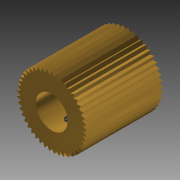
# Autodesk Inventor part: extruder_gear
Saved by Autodesk Inventor 2013 (Build 170138000, 138)
## iProperties
Created: 2015-02-21
Part Number: extruder_gear
Material: 一般
Document SubType Name: Modeling
Designer: Noa Izumi
Density: 1 g/cm^3
Author: Noa Izumi
Autodesk Inventor part; units mm, degrees
ref_plane "YZ Plane" through (0, 0, 0) normal (1, 0, 0) x (0, 1, 0)
ref_plane "XZ Plane" through (0, 0, 0) normal (0, 1, 0) x (-1, 0, 0)
ref_plane "XY Plane" through (0, 0, 0) normal (0, 0, 1) x (1, 0, 0)
sketch "草圖1" plane through (0, 0, 0) normal (0, 1, 0) x (-1, 0, 0)
  circle A0 centre (0, 0) radius 4.75
  line L0 (0, 5.5) -> (0.6495, 4.375)
  line L1 (0.6495, 4.375) -> (-0.6495, 4.375)
  line L2 (-0.6495, 4.375) -> (0, 5.5)
  line L3 (-0.7655, 5.4465) -> (0.0343, 4.4228)
  line L4 (0.0343, 4.4228) -> (-1.2521, 4.242)
  line L5 (-1.2521, 4.242) -> (-0.7655, 5.4465)
  line L6 (-1.516, 5.2869) -> (-0.5816, 4.3846)
  line L7 (-0.5816, 4.3846) -> (-1.8303, 4.0265)
  line L8 (-1.8303, 4.0265) -> (-1.516, 5.2869)
  line L9 (-2.2371, 5.0245) -> (-1.1861, 4.2609)
  line L10 (-1.1861, 4.2609) -> (-2.3728, 3.7326)
  line L11 (-2.3728, 3.7326) -> (-2.2371, 5.0245)
  line L12 (-2.9146, 4.6643) -> (-1.7676, 4.0544)
  line L13 (-1.7676, 4.0544) -> (-2.8692, 3.366)
  line L14 (-2.8692, 3.366) -> (-2.9146, 4.6643)
  line L15 (-3.5353, 4.2132) -> (-2.3146, 3.7689)
  line L16 (-2.3146, 3.7689) -> (-3.3098, 2.9339)
  line L17 (-3.3098, 2.9339) -> (-3.5353, 4.2132)
  line L18 (-4.0873, 3.6802) -> (-2.8166, 3.4101)
  line L19 (-2.8166, 3.4101) -> (-3.6859, 2.4448)
  line L20 (-3.6859, 2.4448) -> (-4.0873, 3.6802)
  line L21 (-4.5597, 3.0756) -> (-3.2638, 2.9849)
  line L22 (-3.2638, 2.9849) -> (-3.9902, 1.908)
  line L23 (-3.9902, 1.908) -> (-4.5597, 3.0756)
  line L24 (-4.9434, 2.411) -> (-3.6475, 2.5017)
  line L25 (-3.6475, 2.5017) -> (-4.217, 1.3341)
  line L26 (-4.217, 1.3341) -> (-4.9434, 2.411)
  line L27 (-5.2308, 1.6996) -> (-3.9602, 1.9697)
  line L28 (-3.9602, 1.9697) -> (-4.3616, 0.7342)
  line L29 (-4.3616, 0.7342) -> (-5.2308, 1.6996)
  line L30 (-5.4164, 0.9551) -> (-4.1957, 1.3994)
  line L31 (-4.1957, 1.3994) -> (-4.4213, 0.1201)
  line L32 (-4.4213, 0.1201) -> (-5.4164, 0.9551)
  line L33 (-5.4966, 0.1919) -> (-4.3497, 0.8018)
  line L34 (-4.3497, 0.8018) -> (-4.395, -0.4964)
  line L35 (-4.395, -0.4964) -> (-5.4966, 0.1919)
  line L36 (-5.4699, -0.5749) -> (-4.4189, 0.1886)
  line L37 (-4.4189, 0.1886) -> (-4.2831, -1.1033)
  line L38 (-4.2831, -1.1033) -> (-5.4699, -0.5749)
  line L39 (-5.3366, -1.3306) -> (-4.4022, -0.4282)
  line L40 (-4.4022, -0.4282) -> (-4.0879, -1.6886)
  line L41 (-4.0879, -1.6886) -> (-5.3366, -1.3306)
  line L42 (-5.0995, -2.0603) -> (-4.2997, -1.0367)
  line L43 (-4.2997, -1.0367) -> (-3.8131, -2.2411)
  line L44 (-3.8131, -2.2411) -> (-5.0995, -2.0603)
  line L45 (-4.7631, -2.75) -> (-4.1136, -1.625)
  line L46 (-4.1136, -1.625) -> (-3.4641, -2.75)
  line L47 (-3.4641, -2.75) -> (-4.7631, -2.75)
  line L48 (-4.3341, -3.3861) -> (-3.8474, -2.1817)
  line L49 (-3.8474, -2.1817) -> (-3.0477, -3.2053)
  line L50 (-3.0477, -3.2053) -> (-4.3341, -3.3861)
  line L51 (-3.8206, -3.9564) -> (-3.5064, -2.6959)
  line L52 (-3.5064, -2.6959) -> (-2.5719, -3.5983)
  line L53 (-2.5719, -3.5983) -> (-3.8206, -3.9564)
  line L54 (-3.2328, -4.4496) -> (-3.097, -3.1577)
  line L55 (-3.097, -3.1577) -> (-2.0461, -3.9212)
  line L56 (-2.0461, -3.9212) -> (-3.2328, -4.4496)
  line L57 (-2.5821, -4.8562) -> (-2.6274, -3.558)
  line L58 (-2.6274, -3.558) -> (-1.4804, -4.1678)
  line L59 (-1.4804, -4.1678) -> (-2.5821, -4.8562)
  line L60 (-1.8811, -5.1683) -> (-2.1067, -3.889)
  line L61 (-2.1067, -3.889) -> (-0.886, -4.3333)
  line L62 (-0.886, -4.3333) -> (-1.8811, -5.1683)
  line L63 (-1.1435, -5.3798) -> (-1.5449, -4.1444)
  line L64 (-1.5449, -4.1444) -> (-0.2743, -4.4144)
  line L65 (-0.2743, -4.4144) -> (-1.1435, -5.3798)
  line L66 (-0.3837, -5.4866) -> (-0.9531, -4.319)
  line L67 (-0.9531, -4.319) -> (0.3428, -4.4097)
  line L68 (0.3428, -4.4097) -> (-0.3837, -5.4866)
  line L69 (0.3837, -5.4866) -> (-0.3428, -4.4097)
  line L70 (-0.3428, -4.4097) -> (0.9531, -4.319)
  line L71 (0.9531, -4.319) -> (0.3837, -5.4866)
  line L72 (1.1435, -5.3798) -> (0.2743, -4.4144)
  line L73 (0.2743, -4.4144) -> (1.5449, -4.1444)
  line L74 (1.5449, -4.1444) -> (1.1435, -5.3798)
  line L75 (1.8811, -5.1683) -> (0.886, -4.3333)
  line L76 (0.886, -4.3333) -> (2.1067, -3.889)
  line L77 (2.1067, -3.889) -> (1.8811, -5.1683)
  line L78 (2.5821, -4.8562) -> (1.4804, -4.1678)
  line L79 (1.4804, -4.1678) -> (2.6274, -3.558)
  line L80 (2.6274, -3.558) -> (2.5821, -4.8562)
  line L81 (3.2328, -4.4496) -> (2.0461, -3.9212)
  line L82 (2.0461, -3.9212) -> (3.097, -3.1577)
  line L83 (3.097, -3.1577) -> (3.2328, -4.4496)
  line L84 (3.8206, -3.9564) -> (2.5719, -3.5983)
  line L85 (2.5719, -3.5983) -> (3.5064, -2.6959)
  line L86 (3.5064, -2.6959) -> (3.8206, -3.9564)
  line L87 (4.3341, -3.3861) -> (3.0477, -3.2053)
  line L88 (3.0477, -3.2053) -> (3.8474, -2.1817)
  line L89 (3.8474, -2.1817) -> (4.3341, -3.3861)
  line L90 (4.7631, -2.75) -> (3.4641, -2.75)
  line L91 (3.4641, -2.75) -> (4.1136, -1.625)
  line L92 (4.1136, -1.625) -> (4.7631, -2.75)
  line L93 (5.0995, -2.0603) -> (3.8131, -2.2411)
  line L94 (3.8131, -2.2411) -> (4.2997, -1.0367)
  line L95 (4.2997, -1.0367) -> (5.0995, -2.0603)
  line L96 (5.3366, -1.3306) -> (4.0879, -1.6886)
  line L97 (4.0879, -1.6886) -> (4.4022, -0.4282)
  line L98 (4.4022, -0.4282) -> (5.3366, -1.3306)
  line L99 (5.4699, -0.5749) -> (4.2831, -1.1033)
  line L100 (4.2831, -1.1033) -> (4.4189, 0.1886)
  line L101 (4.4189, 0.1886) -> (5.4699, -0.5749)
  line L102 (5.4966, 0.1919) -> (4.395, -0.4964)
  line L103 (4.395, -0.4964) -> (4.3497, 0.8018)
  line L104 (4.3497, 0.8018) -> (5.4966, 0.1919)
  line L105 (5.4164, 0.9551) -> (4.4213, 0.1201)
  line L106 (4.4213, 0.1201) -> (4.1957, 1.3994)
  line L107 (4.1957, 1.3994) -> (5.4164, 0.9551)
  line L108 (5.2308, 1.6996) -> (4.3616, 0.7342)
  line L109 (4.3616, 0.7342) -> (3.9602, 1.9697)
  line L110 (3.9602, 1.9697) -> (5.2308, 1.6996)
  line L111 (4.9434, 2.411) -> (4.217, 1.3341)
  line L112 (4.217, 1.3341) -> (3.6475, 2.5017)
  line L113 (3.6475, 2.5017) -> (4.9434, 2.411)
  line L114 (4.5597, 3.0756) -> (3.9902, 1.908)
  line L115 (3.9902, 1.908) -> (3.2638, 2.9849)
  line L116 (3.2638, 2.9849) -> (4.5597, 3.0756)
  line L117 (4.0873, 3.6802) -> (3.6859, 2.4448)
  line L118 (3.6859, 2.4448) -> (2.8166, 3.4101)
  line L119 (2.8166, 3.4101) -> (4.0873, 3.6802)
  line L120 (3.5353, 4.2132) -> (3.3098, 2.9339)
  line L121 (3.3098, 2.9339) -> (2.3146, 3.7689)
  line L122 (2.3146, 3.7689) -> (3.5353, 4.2132)
  line L123 (2.9146, 4.6643) -> (2.8692, 3.366)
  line L124 (2.8692, 3.366) -> (1.7676, 4.0544)
  line L125 (1.7676, 4.0544) -> (2.9146, 4.6643)
  line L126 (2.2371, 5.0245) -> (2.3728, 3.7326)
  line L127 (2.3728, 3.7326) -> (1.1861, 4.2609)
  line L128 (1.1861, 4.2609) -> (2.2371, 5.0245)
  line L129 (1.516, 5.2869) -> (1.8303, 4.0265)
  line L130 (1.8303, 4.0265) -> (0.5816, 4.3846)
  line L131 (0.5816, 4.3846) -> (1.516, 5.2869)
  line L132 (0.7655, 5.4465) -> (1.2521, 4.242)
  line L133 (1.2521, 4.242) -> (-0.0343, 4.4228)
  line L134 (-0.0343, 4.4228) -> (0.7655, 5.4465)
  point P0 (0, 4.75)
  point P1 (-0.6611, 4.7038)
  point P2 (-1.3093, 4.566)
  point P3 (-1.932, 4.3393)
  point P4 (-2.5171, 4.0282)
  point P5 (-3.0532, 3.6387)
  point P6 (-3.5299, 3.1784)
  point P7 (-3.9379, 2.6562)
  point P8 (-4.2693, 2.0823)
  point P9 (-4.5175, 1.4678)
  point P10 (-4.6778, 0.8248)
  point P11 (-4.7471, 0.1658)
  point P12 (-4.724, -0.4965)
  point P13 (-4.6089, -1.1491)
  point P14 (-4.4041, -1.7794)
  point P15 (-4.1136, -2.375)
  point P16 (-3.7431, -2.9244)
  point P17 (-3.2996, -3.4169)
  point P18 (-2.792, -3.8428)
  point P19 (-2.23, -4.194)
  point P20 (-1.6246, -4.4635)
  point P21 (-0.9876, -4.6462)
  point P22 (-0.3313, -4.7384)
  point P23 (0.3313, -4.7384)
  point P24 (0.9876, -4.6462)
  point P25 (1.6246, -4.4635)
  point P26 (2.23, -4.194)
  point P27 (2.792, -3.8428)
  point P28 (3.2996, -3.4169)
  point P29 (3.7431, -2.9244)
  point P30 (4.1136, -2.375)
  point P31 (4.4041, -1.7794)
  point P32 (4.6089, -1.1491)
  point P33 (4.724, -0.4965)
  point P34 (4.7471, 0.1658)
  point P35 (4.6778, 0.8248)
  point P36 (4.5175, 1.4678)
  point P37 (4.2693, 2.0823)
  point P38 (3.9379, 2.6562)
  point P39 (3.5299, 3.1784)
  point P40 (3.0532, 3.6387)
  point P41 (2.5171, 4.0282)
  point P42 (1.932, 4.3393)
  point P43 (1.3093, 4.566)
  point P44 (0.6611, 4.7038)
  dimension "d0" = 9.5
  dimension "d5" = 360
  constraints: 270 end point, 1 coincident, 1 vertical alignment, 325 other
extrude "擠出1" add sketch "草圖1" along normal blind 12
sketch "草圖2" plane through (0, 0, 0) normal (0, -1, 0) x (1, 0, 0)
  point P0 (0, 0)
  point P1 (0, 0)
  constraints: 1 coincident
hole "孔1" at (0, 0, 0) direction (0, 1, 0) diameter 5 end through all
sketch "草圖3" plane through (0, 0, 0) normal (0, 0, 1) x (1, 0, 0)
  point P0 (0, 0)
  point P1 (0, 3)
  dimension "d19" = 3
  measures "d19" distance of point (0, 0) point (0, 3)
hole "孔2" at (0, 3, 0) direction (0, 0, -1) diameter 1.567 end through all thread size "M2x0.4" class "6H" standard "ANSI Metric M Profile"
